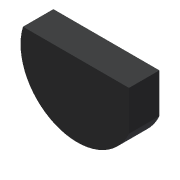
# Autodesk Inventor part: Component_4
Saved by Autodesk Inventor 2022 Beta2 (Build 260130000, 130) ContinuousBuild 0
## iProperties
Shininess: 64.0
Length Units: 11269
Angle Units: 11279
Time Units: 11290
Mass Units: 11283
Length Display Precision: 3
Angle Display Precision: 2
Compacted: True
Part Number: Component_4
Document SubType Name: Modeling
Created: 2004-04-21
Designer: mpaknia
Manufacturer: Standard
Standards Organization: Custom
Density: 1 g/cm^3
Material: Generic
Appearance: Generic
Density: 0.0
Volumn: 0.0
Area: 0.0
PropertySet Name: Model Information
Control State: 0
Master: False
Checked Out: False
Author: mpaknia
Autodesk Inventor part; units mm, degrees
ref_plane "YZ Plane" through (0, 0, 0) normal (1, 0, 0) x (0, 1, 0)
ref_plane "XZ Plane" through (0, 0, 0) normal (0, 1, 0) x (-1, 0, 0)
ref_plane "XY Plane" through (0, 0, 0) normal (0, 0, 1) x (1, 0, 0)
sketch "Sketch2" plane through (0, 0, 0) normal (0, 1, 0) x (-1, 0, 0)
  line L0 (-27.2, 0) -> (20.4, 0) projected
  line L1 (0, 8.6664) -> (0, 28.1819) projected
  line L2 (-17, 11) -> (-17, 24)
  line L3 (-17, 24) -> (17.8478, 24)
  arc A0 (-17, 11) -> (17.8478, 24) centre (0, 18.6364) ccw
  dimension "d1" = 24
  dimension "d2" = 18.6364
  dimension "d3" = 17
  dimension "d4" = 18.6364
  constraints: 4 end point, 2 point on circle, 1 centre point, 1 parallel, 1 perpendicular
  measures "d1" distance between parallel lines of L0 L3
  measures "d2" radius of A0
  measures "d3" distance between parallel lines of L1 L2
  measures "d4" distance from line of L0 A0.centre
extrude "Extrusion1" add sketch "Sketch2" along normal blind 10
body "Solid1"
